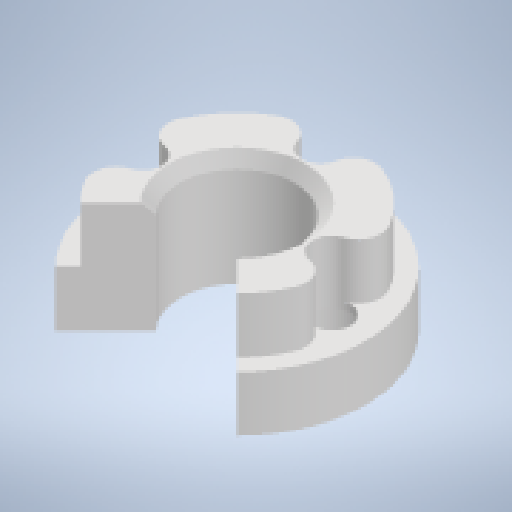
# Autodesk Inventor part: Polea
Saved by Autodesk Inventor 2024 (Build 280153000, 153)
## iProperties
Created: 2025-03-01
Part Number: Polea
Material: Genérico
Document SubType Name: Modeling
Designer: sergi
Density: 1 g/cm^3
Appearance: Valor por defecto
Author: sergi
Autodesk Inventor part; units mm, degrees
ref_plane "YZ Plane" through (0, 0, 0) normal (1, 0, 0) x (0, 1, 0)
ref_plane "XZ Plane" through (0, 0, 0) normal (0, 1, 0) x (-1, 0, 0)
ref_plane "XY Plane" through (0, 0, 0) normal (0, 0, 1) x (1, 0, 0)
sketch "Boceto1" plane through (0, 0, 0) normal (0, 1, 0) x (-1, 0, 0)
  circle A0 centre (0, 0) radius 5.3
  circle A1 centre (0, 0) radius 14
  dimension "d0" = 10.6
  dimension "d1" = 28
  constraints: 2 centre point, 2 coincident
  measures "d0" diameter of A0
  measures "d1" diameter of A1
extrude "Extrusión1" add sketch "Boceto1" along normal blind 10
sketch "Boceto2" plane through (0, 10, 0) normal (0, 1, 0) x (1, 0, 0)
  circle A0 centre (-0.494, 8.0223) radius 1.425 projected
  circle A1 centre (-0.494, 8.0223) radius 1.425 projected
  circle A2 centre (-8.0223, -0.494) radius 1.425 projected
  circle A3 centre (0.494, -8.0223) radius 1.425 projected
  circle A4 centre (8.0223, 0.494) radius 1.425 projected
  circle A5 centre (0, 0) radius 11 projected
  circle A6 centre (0, 0) radius 1.5 projected
  point P0 (0, 0)
hole "Agujero1" at (-0.494, 10, -8.0223) at (8.0223, 10, -0.494) at (0.494, 10, 8.0223) at (-8.0223, 10, 0.494) direction (0, -1, 0) diameter 3.4 end through all
sketch "Boceto3" plane through (0, 0, 0) normal (0, -1, 0) x (1, 0, 0)
  circle A0 centre (-8.0223, 0.494) radius 1.7 projected
  circle A1 centre (0.494, 8.0223) radius 1.7 projected
  circle A2 centre (8.0223, -0.494) radius 1.7 projected
  circle A3 centre (-0.494, -8.0223) radius 1.7 projected
  circle A4 centre (0, 0) radius 14 projected
  circle A5 centre (0, 0) radius 5.3 projected
hole "Agujero2" at (-0.494, 0, -8.0223) at (-8.0223, 0, 0.494) at (0.494, 0, 8.0223) at (8.0223, 0, -0.494) direction (0, 1, 0) diameter 4.5 depth 4 tip angle 118
sketch "Boceto4" plane through (0, 10, 0) normal (0, 1, 0) x (1, 0, 0)
  circle A0 centre (-0.494, 8.0223) radius 1.425 projected
  circle A1 centre (-8.0223, -0.494) radius 1.425 projected
  circle A2 centre (0.494, -8.0223) radius 1.425 projected
  circle A3 centre (8.0223, 0.494) radius 1.425 projected
  circle A4 centre (0, 0) radius 11 projected
  circle A5 centre (0, 0) radius 5 projected
  line L0 (-9.7564, -2.194) -> (-8.0223, -2.194)
  circle A6 centre (-8.0223, -0.494) radius 1.7 projected
  line L1 (-8.0223, 1.206) -> (-9.927, 1.206)
  line L2 (-1.206, -8.0223) -> (-1.206, -9.927)
  line L3 (2.194, -9.7564) -> (2.194, -8.0223)
  line L4 (8.0223, -1.206) -> (9.927, -1.206)
  line L5 (9.7564, 2.194) -> (8.0223, 2.194)
  line L6 (1.206, 8.0223) -> (1.206, 9.927)
  line L7 (-2.194, 9.7564) -> (-2.194, 8.0223)
  arc A7 (-2.194, 9.7564) -> (-9.927, 1.206) centre (0, 0) ccw
  arc A8 (9.7564, 2.194) -> (1.206, 9.927) centre (0, 0) ccw
  arc A9 (-9.7564, -2.194) -> (-1.206, -9.927) centre (0, 0) ccw
  arc A10 (2.194, -9.7564) -> (9.927, -1.206) centre (0, 0) ccw
  circle A11 centre (-0.494, 8.0223) radius 1.425 projected
  circle A12 centre (-8.0223, -0.494) radius 1.425 projected
  circle A13 centre (0.494, -8.0223) radius 1.425 projected
  circle A14 centre (8.0223, 0.494) radius 1.425 projected
  circle A15 centre (0, 0) radius 11 projected
  circle A16 centre (0, 0) radius 1.5 projected
  circle A17 centre (-0.494, 8.0223) radius 1.425 projected
  circle A18 centre (-8.0223, -0.494) radius 1.425 projected
  circle A19 centre (0.494, -8.0223) radius 1.425 projected
  circle A20 centre (8.0223, 0.494) radius 1.425 projected
  circle A21 centre (0, 0) radius 11 projected
  circle A22 centre (0, 0) radius 5 projected
  circle A23 centre (-0.494, 8.0223) radius 1.425 projected
  circle A24 centre (-8.0223, -0.494) radius 1.425 projected
  circle A25 centre (0.494, -8.0223) radius 1.425 projected
  circle A26 centre (8.0223, 0.494) radius 1.425 projected
  circle A27 centre (0, 0) radius 11 projected
  circle A28 centre (0, 0) radius 5 projected
  circle A29 centre (0.494, -8.0223) radius 1.7 projected
  circle A30 centre (8.0223, 0.494) radius 1.7 projected
  circle A31 centre (-0.494, 8.0223) radius 1.7 projected
  circle A32 centre (0, 0) radius 14 projected
  dimension "d21" = 360
  constraints: 16 end point, 10 point on circle, 4 centre point, 3 coincident, 2 horizontal, 2 tangent, 25 other
extrude "Extrusión2" cut sketch "Boceto4" against normal blind 5 contours A4 | A32
fillet "Empalme1" radius 2 8 edges at (-9.7564, 7.5, 2.194) (-9.927, 7.5, -1.206) (-2.194, 7.5, -9.7564) (1.206, 7.5, -9.927) (-1.206, 7.5, 9.927) (2.194, 7.5, 9.7564) (9.927, 7.5, 1.206) (9.7564, 7.5, -2.194)
chamfer "Chaflán1" distance 1 angle 45 1 edges at (5.3, 10, 0)
sketch "Boceto5" plane through (0, 0, 0) normal (0, -1, 0) x (1, 0, 0)
  arc A0 (2.116, 7.5132) -> (-1.1782, 7.716) centre (0.494, 8.0223) ccw projected
  arc A1 (-1.1782, 7.716) -> (-3.9318, 9.1946) centre (-3.1455, 7.3557) ccw projected
  arc A2 (-3.9318, 9.1946) -> (-8.6428, 5.0302) centre (0, 0) ccw projected
  arc A3 (-8.6428, 5.0302) -> (-7.5132, 2.116) centre (-6.9142, 4.0242) ccw projected
  arc A4 (-7.5132, 2.116) -> (-7.716, -1.1782) centre (-8.0223, 0.494) ccw projected
  arc A5 (-7.716, -1.1782) -> (-9.1946, -3.9318) centre (-7.3557, -3.1455) ccw projected
  arc A6 (-9.1946, -3.9318) -> (-5.0302, -8.6428) centre (0, 0) ccw projected
  arc A7 (-5.0302, -8.6428) -> (-2.116, -7.5132) centre (-4.0242, -6.9142) ccw projected
  arc A8 (-2.116, -7.5132) -> (1.1782, -7.716) centre (-0.494, -8.0223) ccw projected
  arc A9 (1.1782, -7.716) -> (3.9318, -9.1946) centre (3.1455, -7.3557) ccw projected
  arc A10 (3.9318, -9.1946) -> (8.6428, -5.0302) centre (0, 0) ccw projected
  arc A11 (8.6428, -5.0302) -> (7.5132, -2.116) centre (6.9142, -4.0242) ccw projected
  arc A12 (7.5132, -2.116) -> (7.716, 1.1782) centre (8.0223, -0.494) ccw projected
  arc A13 (7.716, 1.1782) -> (9.1946, 3.9318) centre (7.3557, 3.1455) ccw projected
  arc A14 (9.1946, 3.9318) -> (5.0302, 8.6428) centre (0, 0) ccw projected
  arc A15 (5.0302, 8.6428) -> (2.116, 7.5132) centre (4.0242, 6.9142) ccw projected
  circle A16 centre (0, 0) radius 14 projected
  line L0 (0.494, 8.0223) -> (-0.494, -8.0223)
  line L1 (0, 0) -> (7.2809, 16.7261)
  line L2 (0, 0) -> (19.4725, 5.7593)
  point P0 (13.4251, 3.9707)
  point P1 (5.5878, 12.8365)
  dimension "d40" = 20
  dimension "d41" = 50
  constraints: 6 end point
  measures "d40" angle of L0 L1
  measures "d41" angle of L1 L2
extrude "Extrusión3" cut sketch "Boceto5" against normal through all contours L1 A16 L2 A13 A14 A15 | A15 A14 A13 L2 L1
sketch "Boceto6" plane through (0, 10, 0) normal (0, 1, 0) x (1, 0, 0)
  arc A0 (13.4251, -3.9707) -> (5.5878, -12.8365) centre (0, 0) ccw projected
  arc A1 (2.116, -7.5132) -> (3.878, -8.9089) centre (4.0242, -6.9142) ccw projected
  arc A2 (-1.1782, -7.716) -> (2.116, -7.5132) centre (0.494, -8.0223) ccw projected
  arc A3 (-3.9318, -9.1946) -> (-1.1782, -7.716) centre (-3.1455, -7.3557) ccw projected
  arc A4 (-8.6428, -5.0302) -> (-3.9318, -9.1946) centre (0, 0) ccw projected
  arc A5 (-7.5132, -2.116) -> (-8.6428, -5.0302) centre (-6.9142, -4.0242) ccw projected
  arc A6 (-7.716, 1.1782) -> (-7.5132, -2.116) centre (-8.0223, -0.494) ccw projected
  arc A7 (-9.1946, 3.9318) -> (-7.716, 1.1782) centre (-7.3557, 3.1455) ccw projected
  arc A8 (-5.0302, 8.6428) -> (-9.1946, 3.9318) centre (0, 0) ccw projected
  arc A9 (-2.116, 7.5132) -> (-5.0302, 8.6428) centre (-4.0242, 6.9142) ccw projected
  arc A10 (1.1782, 7.716) -> (-2.116, 7.5132) centre (-0.494, 8.0223) ccw projected
  arc A11 (3.9318, 9.1946) -> (1.1782, 7.716) centre (3.1455, 7.3557) ccw projected
  arc A12 (8.6428, 5.0302) -> (3.9318, 9.1946) centre (0, 0) ccw projected
  arc A13 (7.5132, 2.116) -> (8.6428, 5.0302) centre (6.9142, 4.0242) ccw projected
  arc A14 (7.716, -1.1782) -> (7.5132, 2.116) centre (8.0223, 0.494) ccw projected
  arc A15 (9.3173, -2.7557) -> (7.716, -1.1782) centre (7.3557, -3.1455) ccw projected
  circle A16 centre (0, 0) radius 13
  arc A17 (6.0413, -1.7868) -> (2.5145, -5.7764) centre (0, 0) ccw projected
  line L0 (4.1548, -8.9099) -> (-1.0984, 2.3556) projected
  circle A18 centre (0, 0) radius 6.15
  arc A19 (6.0413, -1.7868) -> (2.5145, -5.7764) centre (0, 0) ccw projected
  arc A20 (9.3173, -2.7557) -> (7.716, -1.1782) centre (7.3557, -3.1455) ccw projected
  arc A21 (7.5132, 2.116) -> (7.716, -1.1782) centre (8.0223, 0.494) ccw projected
  arc A22 (7.5132, 2.116) -> (8.6428, 5.0302) centre (6.9142, 4.0242) ccw projected
  arc A23 (8.6428, 5.0302) -> (3.9318, 9.1946) centre (0, 0) ccw projected
  arc A24 (3.9318, 9.1946) -> (1.1782, 7.716) centre (3.1455, 7.3557) ccw projected
  arc A25 (-2.116, 7.5132) -> (1.1782, 7.716) centre (-0.494, 8.0223) ccw projected
  arc A26 (-2.116, 7.5132) -> (-5.0302, 8.6428) centre (-4.0242, 6.9142) ccw projected
  arc A27 (-5.0302, 8.6428) -> (-9.1946, 3.9318) centre (0, 0) ccw projected
  arc A28 (-9.1946, 3.9318) -> (-7.716, 1.1782) centre (-7.3557, 3.1455) ccw projected
  arc A29 (-7.5132, -2.116) -> (-7.716, 1.1782) centre (-8.0223, -0.494) ccw projected
  arc A30 (-7.5132, -2.116) -> (-8.6428, -5.0302) centre (-6.9142, -4.0242) ccw projected
  arc A31 (-8.6428, -5.0302) -> (-3.9318, -9.1946) centre (0, 0) ccw projected
  arc A32 (-3.9318, -9.1946) -> (-1.1782, -7.716) centre (-3.1455, -7.3557) ccw projected
  arc A33 (2.116, -7.5132) -> (-1.1782, -7.716) centre (0.494, -8.0223) ccw projected
  arc A34 (2.116, -7.5132) -> (3.878, -8.9089) centre (4.0242, -6.9142) ccw projected
  line L1 (3.878, -8.9089) -> (2.5145, -5.7764) projected
  line L2 (6.0413, -1.7868) -> (9.3173, -2.7557) projected
  line L3 (5.5878, -12.8365) -> (3.878, -8.9089) projected
  line L4 (9.3173, -2.7557) -> (13.4251, -3.9707) projected
  point P0 (5.494, -11.782)
  point P1 (-6.15, 0)
  point P2 (-6.15, 0)
  point P3 (5.8975, -1.7443)
  point P4 (13, 0)
  point P5 (2.116, -7.5132)
  point P6 (-1.1782, -7.716)
  point P7 (1.1782, 7.716)
  point P8 (7.716, -1.1782)
  point P9 (2.4546, -5.6389)
  point P10 (5.8975, -1.7443)
  point P11 (-1.1782, -7.716)
  point P12 (2.116, -7.5132)
  point P13 (3.878, -8.9089)
  point P14 (3.7118, -8.5269)
  point P15 (1.0369, -6.2141)
  point P16 (9.3173, -2.7557)
  point P17 (7.716, -1.1782)
  point P18 (1.1782, 7.716)
  constraints: 2 coincident, 7 other
extrude "Extrusión4" [suppressed]
chamfer "Chaflán2" [suppressed]
chamfer "Chaflán3" distance 5 distance2 4 1 edges at (-10.4892, 5, -9.2724) measured on face at (13.7052, 3.3333, 2.858)
